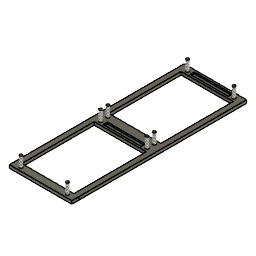
bus (Autodesk Fusion 360 archive; units mm, degrees)
design "ramka na 2 ekrany"
part number: 2026-03-25-11-53-01-845
Autodesk Fusion 360 part; units mm, degrees
note: some values were not read from the file. Chosen so that the rebuilt part matches the saved one: which bodies a step acts on; which face or edge a step refers to; how an offset face is resized. Set by a fixed rule: which sketch regions a step uses.
sketch "Sketch1" plane through (0, 0, 0) normal (0, 0, 1) x (1, 0, 0)
  line L0 (45, 35) -> (-45, 35)
  line L1 (-45, 35) -> (-45, -35)
  line L2 (-45, -35) -> (45, -35)
  line L3 (45, -35) -> (45, 35)
  line L4 (45, 35) -> (-45, -35) construction
  line L5 (-45, 35) -> (45, -35) construction
  line L6 (34.75, 25.0029) -> (-34.75, 25.0029)
  line L7 (-34.75, 25.0029) -> (-34.75, -24.9971)
  line L8 (-34.75, -24.9971) -> (34.75, -24.9971)
  line L9 (34.75, -24.9971) -> (34.75, 25.0029)
  line L10 (34.75, 25.0029) -> (-34.75, -24.9971) construction
  line L11 (-34.75, 25.0029) -> (34.75, -24.9971) construction
  point P0 (0, 0.0029)
  dimension "d1" = 90
  dimension "d2" = 70
  dimension "d3" = 69.5
  dimension "d4" = 50
  constraint horizontal L0
  constraint perpendicular L0 L1
  constraint parallel L0 L2
  constraint parallel L1 L3
  constraint coincident L4 origin
  constraint coincident L5 origin
  constraint horizontal L6
  constraint perpendicular L6 L7
  constraint parallel L6 L8
  constraint parallel L7 L9
  constraint coincident L10 P0
  constraint coincident L11 P0
  measures "d1" distance of L0.start L0.end
  measures "d2" distance of L0.start L2.end
  measures "d3" distance of L6.start L6.end
  measures "d4" distance of L6.start L8.end
extrude "Extrude1" add sketch "Sketch1" along normal blind 3 contours L0 L1 L2 L3 | L6 L7 L8 L9 makes body 1
extrude "Extrude2" cut sketch "Sketch1" along normal blind 42 contours L6 L7 L8 L9 bodies 1
ref_plane "WorkPlane1" through (0, 0, 3) normal (0, 0, 1) x (1, 0, 0)
sketch "Sketch2" plane through (0, 0, 3) normal (0, 0, 1) x (1, 0, 0)
  line L0 (38.25, 22.5) -> (38.25, 22.8)
  line L1 (38.25, 22.8) -> (38.25, 27.2)
  line L2 (38.25, 27.2) -> (38.25, -28)
  line L3 (34.7, 25) -> (34.8, 25)
  line L4 (38.25, 25) -> (38.25, 23.8)
  line L5 (34.7, -25) -> (40.2, -25)
  line L6 (38.25, -25) -> (38.25, -23.8)
  circle A0 centre (38.2495, -22.3) radius 1.5
  line L7 (34.8, 25) -> (39.15, 25)
  line L8 (38.25, 25) -> (38.25, 23.8)
  circle A1 centre (38.25, 22.3) radius 1.5
  line L9 (-34, -25) -> (-44, -25)
  line L10 (-22, 25) -> (-43.5908, 25)
  line L11 (-34.75, 25) -> (-38.25, 25)
  line L12 (-38.25, 25) -> (-38.25, -25)
  line L13 (-38.25, -25) -> (-38.25, -23.8)
  circle A2 centre (-38.25, -22.3041) radius 1.5
  line L14 (-38.25, 25) -> (-38.25, 23.8)
  circle A3 centre (-38.25, 22.2805) radius 1.5
  dimension "d13" = 1.2
  dimension "d14" = 3
  dimension "d15" = 1.2
  dimension "d16" = 3
  dimension "d17" = 3.5
  dimension "d18" = 1.2
  dimension "d19" = 3
  dimension "d20" = 1.2
  dimension "d21" = 3
  constraint perpendicular L2 L3
  constraint midpoint L1 L4.start
  constraint perpendicular L2 L5
  constraint coincident L5 L6.start
  constraint coincident L2 L6.start
  constraint perpendicular L5 L6
  constraint coincident L6.end A0
  constraint parallel L3 L7
  constraint coincident L1 A1.centre
  constraint horizontal L9
  constraint horizontal L10
  constraint coincident L10 L11.start
  constraint parallel L10 L11
  constraint coincident L9 L12.end
  constraint perpendicular L9 L12
  constraint perpendicular L9 L13
  constraint coincident L12 A2.centre
  constraint perpendicular L10 L14
  constraint coincident L12 A3.centre
  measures "d13" distance of L6.start L6.end
  measures "d14" diameter of A0
  measures "d15" distance of L4.start L4.end
  measures "d16" diameter of A1
  measures "d17" distance of L11.start L11.end
  measures "d18" distance of L12.end L13.end
  measures "d19" diameter of A2
  measures "d20" distance of L11.end L14.end
  measures "d21" diameter of A3
extrude "Extrude3" add sketch "Sketch2" along normal blind 10 separate body contours L12 A3 | L12 A3 makes body 2
thread "Thread1" "ISO Metric profile 3.0 M3x0.5 M3x0.5 6g" major diameter 2.927 minor diameter 2.3555 pitch 0.5 angle 60 resizes the face on face at (-37.0709, 23.2078, 9.6667) on bodies 2
extrude "Extrude4" add sketch "Sketch2" along normal blind 10 separate body contours L0 L1 L2 A1 | L0 L1 L2 A1 | L2 A0 | L2 A0 | L12 L13 A2 | L12 L13 A2 makes body 3 at (-37.9895, -23.7813, 9.6667) makes body 4 at (37.5652, -20.9652, 9.6667) makes body 5 at (37.5657, 23.6348, 9.6667)
thread "Thread2" "ISO Metric profile 3.0 M3x0.5 M3x0.5 6g" major diameter 2.927 minor diameter 2.3555 pitch 0.5 angle 60 resizes the face on face at (-37.9895, -23.7813, 9.6667) on face at (37.5652, -20.9652, 9.6667) on face at (37.5657, 23.6348, 9.6667) on bodies 3 4 5
sketch "Sketch3" plane through (0, 0, 0) normal (0, 0, 1) x (1, 0, 0)
  line L0 (-2.8868, 5) -> (-5.7735, 0)
  line L1 (-5.7735, 0) -> (-2.8868, -5)
  line L2 (-2.8868, -5) -> (2.8868, -5)
  line L3 (2.8868, -5) -> (5.7735, 0)
  line L4 (5.7735, 0) -> (2.8868, 5)
  line L5 (2.8868, 5) -> (-2.8868, 5)
  circle A0 centre (0, 0) radius 1.5
  dimension "d30" = 5
  dimension "d31" = 3
  constraint coincident A0.centre origin
  measures "d30" distance of A0.centre L5
  measures "d31" diameter of A0
sketch "Sketch4" plane through (0, 0, 3) normal (0, 0, 1) x (1, 0, 0)
  line L0 (34.75, 0) -> (38.75, 0)
  line L1 (42.75, 0) -> (42.75, -18.25)
  line L2 (42.75, -18.25) -> (38.75, -18.25)
  line L3 (38.75, -18.25) -> (38.75, 0)
  line L4 (38.75, 0) -> (38.75, 18.25)
  line L5 (38.75, 18.25) -> (42.75, 18.25)
  line L6 (42.75, 18.25) -> (42.75, 0)
  dimension "d37" = 4
  dimension "d38" = 18.25
  dimension "d39" = 4
  dimension "d40" = 4
  dimension "d41" = 18.25
  constraint horizontal L0
  constraint vertical L1
  constraint horizontal L2
  constraint vertical L3
  constraint vertical L4
  constraint horizontal L5
  constraint vertical L6
  measures "d37" distance of L0.start L0.end
  measures "d38" distance of L0.end L2.end
  measures "d39" distance of L0.end L1.start
  measures "d40" distance of L1.start L0.end
  measures "d41" distance of L1.start L5.end
extrude "Extrude6" cut sketch "Sketch4" against normal blind 1.5 bodies 1
combine "Combine1" operation add target body 1 tool bodies 2 3 5 4
move_body "Move1" bodies 1 to x (0, 1, 0) y (0, 0, 1) z (1, 0, 0) at (-45, 10, 35)
move_body "Move2" bodies 1 to x (0, 0, 1) y (0, 1, 0) z (-1, 0, 0) at (6.0688, 0, 90.0688)
move_body "Move3" bodies 1 to x (1, 0, 0) y (0, 1, 0) z (0, 0, 1) at (0, 0, -45)
extrude "Extrude7" cut 1 faces at (-22.8478, 48.75, 2.0688) along direction (0, -1, 0) blind 2 on bodies 1 bodies 1
extrude "Extrude8" add 1 faces at (-35.0145, 52.75, 2.0688) along direction (0, -1, 0) blind 1.5 on bodies 1 bodies 1
ref_plane "WorkPlane2" through (-28.9312, 10, 3.0688) normal (0, 0, 1) x (0, 1, 0)
sketch "Sketch5" plane through (0, 0, 3.0688) normal (0, 0, 1) x (1, 0, 0)
  line L0 (-53.9341, 44.75) -> (-3.9341, 44.75)
  line L1 (-3.9341, -24.75) -> (-53.9341, -24.75)
  line L2 (-3.9341, 44.75) -> (-3.9341, -24.75)
  line L3 (-53.9341, -24.75) -> (-53.9341, 44.75)
  line L4 (-31.0518, 51.75) -> (-58.9341, 51.75)
  line L5 (-58.9341, 51.75) -> (-58.9341, 25.022)
  line L6 (-58.9341, 25.022) -> (-58.9341, -31)
  line L7 (-58.9341, -31) -> (-58.9341, -31.75)
  line L8 (-58.9341, -31.75) -> (-30.0627, -31.75)
  line L9 (-30.0627, -31.75) -> (1, -31.75)
  line L10 (1, -31.75) -> (4, -31.75)
  line L11 (1.0659, -24.75) -> (1, -31.75)
  line L12 (1.0659, -24.75) -> (1.0659, 24.1629)
  line L13 (1.0659, 44.75) -> (1.0659, 24.1629)
  line L14 (-31.0518, 51.75) -> (1.0659, 51.75)
  line L15 (1.0659, 51.75) -> (1.0659, 44.75)
  dimension "d54" = 5
  dimension "d55" = 5
  measures "d54" distance of L1.start L11.start
  measures "d55" distance of L0.end L13.start
split "Split1" by curves path "Sketch5" along L11 L12 L13 L15 L14 L4 L5 L6 L7 L8 L9 bodies 1 makes body 6 at (4.4012, 14.721, 3.0688)
delete_body "RemoveBody1" bodies 6
extrude "Extrude9" add 1 faces at (-35.0145, 51.25, 2.0688) along direction (0, -1, 0) blind 0.5 on bodies 1 bodies 1
copy_body "CopyPasteBodies1" bodies 1 makes body 7
move_body "Move4" bodies 7 to x (1, 0, 0) y (0, 1, 0) z (0, 0, 1) at (0, 83.5, 0)
ref_plane "WorkPlane3" through (1.0659, 13.5, 1.5688) normal (1, 0, 0) x (0, 1, 0)
sketch "Sketch6" plane through (1.0659, 0, 0) normal (1, 0, 0) x (0, 1, 0)
  line L0 (51.75, 3.0688) -> (-24.75, 3.0688)
  line L1 (-24.75, 3.0688) -> (-24.75, 0.0688)
  line L2 (-24.75, 0.0688) -> (51.75, 0.0688)
  line L3 (51.75, 0.0688) -> (51.75, 3.0688)
  line L4 (-31.75, 3.0688) -> (135.25, 3.0688)
  line L5 (135.25, 3.0688) -> (135.25, 0.0688)
  line L6 (135.25, 0.0688) -> (-31.75, 0.0688)
  line L7 (-31.75, 0.0688) -> (-31.75, 3.0688)
  point P0 (-31.75, 3.0688)
  point P1 (135.25, 0.0688)
  constraint horizontal L4
  constraint vertical L5
  constraint horizontal L6
  constraint vertical L7
  constraint coincident P1 L5.end
  constraint coincident P0 L4.start
extrude "Extrude10" add sketch "Sketch6" against normal blind 2 contours L3 L4 L5 L6 bodies 1 7
extrude "Extrude11" add 1 faces at (-38.9341, 135.25, 2.0688) along direction (0, 1, 0) blind 1 on bodies 1 bodies 1

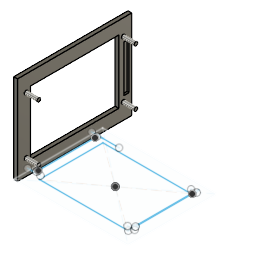
design "ekran TFT"
part number: 2026-03-25-11-53-01-845
Autodesk Fusion 360 part; units mm, degrees
sketch "Sketch1" plane through (0, 0, 0) normal (0, 0, 1) x (1, 0, 0)
  line L0 (45, 35) -> (-45, 35)
  line L1 (-45, 35) -> (-45, -35)
  line L2 (-45, -35) -> (45, -35)
  line L3 (45, -35) -> (45, 35)
  line L4 (45, 35) -> (-45, -35) construction
  line L5 (-45, 35) -> (45, -35) construction
  line L6 (34.75, 25.0029) -> (-34.75, 25.0029)
  line L7 (-34.75, 25.0029) -> (-34.75, -24.9971)
  line L8 (-34.75, -24.9971) -> (34.75, -24.9971)
  line L9 (34.75, -24.9971) -> (34.75, 25.0029)
  line L10 (34.75, 25.0029) -> (-34.75, -24.9971) construction
  line L11 (-34.75, 25.0029) -> (34.75, -24.9971) construction
  point P0 (0, 0.0029)
  dimension "d1" = 90
  dimension "d2" = 70
  dimension "d3" = 69.5
  dimension "d4" = 50
  constraint horizontal L0
  constraint perpendicular L0 L1
  constraint parallel L0 L2
  constraint parallel L1 L3
  constraint coincident L4 origin
  constraint coincident L5 origin
  constraint horizontal L6
  constraint perpendicular L6 L7
  constraint parallel L6 L8
  constraint parallel L7 L9
  constraint coincident L10 P0
  constraint coincident L11 P0
  measures "d1" distance of L0.start L0.end
  measures "d2" distance of L0.start L2.end
  measures "d3" distance of L6.start L6.end
  measures "d4" distance of L6.start L8.end
extrude "Extrude1" add sketch "Sketch1" along normal blind 3 contours L0 L1 L2 L3 | L6 L7 L8 L9 makes body 1
extrude "Extrude2" cut sketch "Sketch1" along normal blind 42 contours L6 L7 L8 L9 bodies 1
ref_plane "WorkPlane1" through (0, 0, 3) normal (0, 0, 1) x (1, 0, 0)
sketch "Sketch2" plane through (0, 0, 3) normal (0, 0, 1) x (1, 0, 0)
  line L0 (38.25, 22.5) -> (38.25, 22.8)
  line L1 (38.25, 22.8) -> (38.25, 27.2)
  line L2 (38.25, 27.2) -> (38.25, -28)
  line L3 (34.7, 25) -> (34.8, 25)
  line L4 (38.25, 25) -> (38.25, 23.8)
  line L5 (34.7, -25) -> (40.2, -25)
  line L6 (38.25, -25) -> (38.25, -23.8)
  circle A0 centre (38.2495, -22.3) radius 1.5
  line L7 (34.8, 25) -> (39.15, 25)
  line L8 (38.25, 25) -> (38.25, 23.8)
  circle A1 centre (38.25, 22.3) radius 1.5
  line L9 (-34, -25) -> (-44, -25)
  line L10 (-22, 25) -> (-43.5908, 25)
  line L11 (-34.75, 25) -> (-38.25, 25)
  line L12 (-38.25, 25) -> (-38.25, -25)
  line L13 (-38.25, -25) -> (-38.25, -23.8)
  circle A2 centre (-38.25, -22.3041) radius 1.5
  line L14 (-38.25, 25) -> (-38.25, 23.8)
  circle A3 centre (-38.25, 22.2805) radius 1.5
  dimension "d13" = 1.2
  dimension "d14" = 3
  dimension "d15" = 1.2
  dimension "d16" = 3
  dimension "d17" = 3.5
  dimension "d18" = 1.2
  dimension "d19" = 3
  dimension "d20" = 1.2
  dimension "d21" = 3
  constraint perpendicular L2 L3
  constraint midpoint L1 L4.start
  constraint perpendicular L2 L5
  constraint coincident L5 L6.start
  constraint coincident L2 L6.start
  constraint perpendicular L5 L6
  constraint coincident L6.end A0
  constraint parallel L3 L7
  constraint coincident L1 A1.centre
  constraint horizontal L9
  constraint horizontal L10
  constraint coincident L10 L11.start
  constraint parallel L10 L11
  constraint coincident L9 L12.end
  constraint perpendicular L9 L12
  constraint perpendicular L9 L13
  constraint coincident L12 A2.centre
  constraint perpendicular L10 L14
  constraint coincident L12 A3.centre
  measures "d13" distance of L6.start L6.end
  measures "d14" diameter of A0
  measures "d15" distance of L4.start L4.end
  measures "d16" diameter of A1
  measures "d17" distance of L11.start L11.end
  measures "d18" distance of L12.end L13.end
  measures "d19" diameter of A2
  measures "d20" distance of L11.end L14.end
  measures "d21" diameter of A3
extrude "Extrude3" add sketch "Sketch2" along normal blind 10 separate body contours L12 A3 | L12 A3 makes body 2
thread "Thread1" "ISO Metric profile 3.0 M3x0.5 M3x0.5 6g" major diameter 2.927 minor diameter 2.3555 pitch 0.5 angle 60 resizes the face on face at (-37.0709, 23.2078, 9.6667) on bodies 2
extrude "Extrude4" add sketch "Sketch2" along normal blind 10 separate body contours L0 L1 L2 A1 | L0 L1 L2 A1 | L2 A0 | L2 A0 | L12 L13 A2 | L12 L13 A2 makes body 3 at (-37.9895, -23.7813, 9.6667) makes body 4 at (37.5652, -20.9652, 9.6667) makes body 5 at (37.5657, 23.6348, 9.6667)
thread "Thread2" "ISO Metric profile 3.0 M3x0.5 M3x0.5 6g" major diameter 2.927 minor diameter 2.3555 pitch 0.5 angle 60 resizes the face on face at (-37.9895, -23.7813, 9.6667) on face at (37.5652, -20.9652, 9.6667) on face at (37.5657, 23.6348, 9.6667) on bodies 3 4 5
sketch "Sketch3" plane through (0, 0, 0) normal (0, 0, 1) x (1, 0, 0)
  line L0 (-2.8868, 5) -> (-5.7735, 0)
  line L1 (-5.7735, 0) -> (-2.8868, -5)
  line L2 (-2.8868, -5) -> (2.8868, -5)
  line L3 (2.8868, -5) -> (5.7735, 0)
  line L4 (5.7735, 0) -> (2.8868, 5)
  line L5 (2.8868, 5) -> (-2.8868, 5)
  circle A0 centre (0, 0) radius 1.5
  dimension "d30" = 5
  dimension "d31" = 3
  constraint coincident A0.centre origin
  measures "d30" distance of A0.centre L5
  measures "d31" diameter of A0
sketch "Sketch4" plane through (0, 0, 3) normal (0, 0, 1) x (1, 0, 0)
  line L0 (34.75, 0) -> (38.75, 0)
  line L1 (42.75, 0) -> (42.75, -18.25)
  line L2 (42.75, -18.25) -> (38.75, -18.25)
  line L3 (38.75, -18.25) -> (38.75, 0)
  line L4 (38.75, 0) -> (38.75, 18.25)
  line L5 (38.75, 18.25) -> (42.75, 18.25)
  line L6 (42.75, 18.25) -> (42.75, 0)
  dimension "d37" = 4
  dimension "d38" = 18.25
  dimension "d39" = 4
  dimension "d40" = 4
  dimension "d41" = 18.25
  constraint horizontal L0
  constraint vertical L1
  constraint horizontal L2
  constraint vertical L3
  constraint vertical L4
  constraint horizontal L5
  constraint vertical L6
  measures "d37" distance of L0.start L0.end
  measures "d38" distance of L0.end L2.end
  measures "d39" distance of L0.end L1.start
  measures "d40" distance of L1.start L0.end
  measures "d41" distance of L1.start L5.end
extrude "Extrude6" cut sketch "Sketch4" against normal blind 1.5 bodies 1
combine "Combine1" operation add target body 1 tool bodies 2 3 5 4
move_body "Move1" bodies 1 to x (0, 1, 0) y (0, 0, 1) z (1, 0, 0) at (-45, 10, 35)

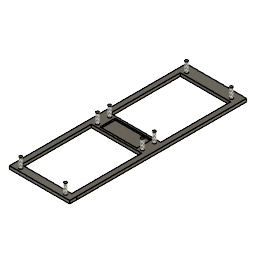
design "ramka wersja 4327643276"
part number: 2026-03-25-11-53-01-845
Autodesk Fusion 360 part; units mm, degrees
sketch "Sketch1" plane through (0, 0, 0) normal (0, 0, 1) x (1, 0, 0)
  line L0 (45, 35) -> (-45, 35)
  line L1 (-45, 35) -> (-45, -35)
  line L2 (-45, -35) -> (45, -35)
  line L3 (45, -35) -> (45, 35)
  line L4 (45, 35) -> (-45, -35) construction
  line L5 (-45, 35) -> (45, -35) construction
  line L6 (34.75, 25.0029) -> (-34.75, 25.0029)
  line L7 (-34.75, 25.0029) -> (-34.75, -24.9971)
  line L8 (-34.75, -24.9971) -> (34.75, -24.9971)
  line L9 (34.75, -24.9971) -> (34.75, 25.0029)
  line L10 (34.75, 25.0029) -> (-34.75, -24.9971) construction
  line L11 (-34.75, 25.0029) -> (34.75, -24.9971) construction
  point P0 (0, 0.0029)
  dimension "d1" = 90
  dimension "d2" = 70
  dimension "d3" = 69.5
  dimension "d4" = 50
  constraint horizontal L0
  constraint perpendicular L0 L1
  constraint parallel L0 L2
  constraint parallel L1 L3
  constraint coincident L4 origin
  constraint coincident L5 origin
  constraint horizontal L6
  constraint perpendicular L6 L7
  constraint parallel L6 L8
  constraint parallel L7 L9
  constraint coincident L10 P0
  constraint coincident L11 P0
  measures "d1" distance of L0.start L0.end
  measures "d2" distance of L0.start L2.end
  measures "d3" distance of L6.start L6.end
  measures "d4" distance of L6.start L8.end
extrude "Extrude1" add sketch "Sketch1" along normal blind 3 contours L0 L1 L2 L3 | L6 L7 L8 L9 makes body 1
extrude "Extrude2" cut sketch "Sketch1" along normal blind 42 contours L6 L7 L8 L9 bodies 1
ref_plane "WorkPlane1" through (0, 0, 3) normal (0, 0, 1) x (1, 0, 0)
sketch "Sketch2" plane through (0, 0, 3) normal (0, 0, 1) x (1, 0, 0)
  line L0 (38.25, 22.5) -> (38.25, 22.8)
  line L1 (38.25, 22.8) -> (38.25, 27.2)
  line L2 (38.25, 27.2) -> (38.25, -28)
  line L3 (34.7, 25) -> (34.8, 25)
  line L4 (38.25, 25) -> (38.25, 23.8)
  line L5 (34.7, -25) -> (40.2, -25)
  line L6 (38.25, -25) -> (38.25, -23.8)
  circle A0 centre (38.2495, -22.3) radius 1.5
  line L7 (34.8, 25) -> (39.15, 25)
  line L8 (38.25, 25) -> (38.25, 23.8)
  circle A1 centre (38.25, 22.3) radius 1.5
  line L9 (-34, -25) -> (-44, -25)
  line L10 (-22, 25) -> (-43.5908, 25)
  line L11 (-34.75, 25) -> (-38.25, 25)
  line L12 (-38.25, 25) -> (-38.25, -25)
  line L13 (-38.25, -25) -> (-38.25, -23.8)
  circle A2 centre (-38.25, -22.3041) radius 1.5
  line L14 (-38.25, 25) -> (-38.25, 23.8)
  circle A3 centre (-38.25, 22.2805) radius 1.5
  dimension "d13" = 1.2
  dimension "d14" = 3
  dimension "d15" = 1.2
  dimension "d16" = 3
  dimension "d17" = 3.5
  dimension "d18" = 1.2
  dimension "d19" = 3
  dimension "d20" = 1.2
  dimension "d21" = 3
  constraint perpendicular L2 L3
  constraint midpoint L1 L4.start
  constraint perpendicular L2 L5
  constraint coincident L5 L6.start
  constraint coincident L2 L6.start
  constraint perpendicular L5 L6
  constraint coincident L6.end A0
  constraint parallel L3 L7
  constraint coincident L1 A1.centre
  constraint horizontal L9
  constraint horizontal L10
  constraint coincident L10 L11.start
  constraint parallel L10 L11
  constraint coincident L9 L12.end
  constraint perpendicular L9 L12
  constraint perpendicular L9 L13
  constraint coincident L12 A2.centre
  constraint perpendicular L10 L14
  constraint coincident L12 A3.centre
  measures "d13" distance of L6.start L6.end
  measures "d14" diameter of A0
  measures "d15" distance of L4.start L4.end
  measures "d16" diameter of A1
  measures "d17" distance of L11.start L11.end
  measures "d18" distance of L12.end L13.end
  measures "d19" diameter of A2
  measures "d20" distance of L11.end L14.end
  measures "d21" diameter of A3
extrude "Extrude3" add sketch "Sketch2" along normal blind 10 separate body contours L12 A3 | L12 A3 makes body 2
thread "Thread1" "ISO Metric profile 3.0 M3x0.5 M3x0.5 6g" major diameter 2.927 minor diameter 2.3555 pitch 0.5 angle 60 resizes the face on face at (-37.0709, 23.2078, 9.6667) on bodies 2
extrude "Extrude4" add sketch "Sketch2" along normal blind 10 separate body contours L0 L1 L2 A1 | L0 L1 L2 A1 | L2 A0 | L2 A0 | L12 L13 A2 | L12 L13 A2 makes body 3 at (-37.9895, -23.7813, 9.6667) makes body 4 at (37.5652, -20.9652, 9.6667) makes body 5 at (37.5657, 23.6348, 9.6667)
thread "Thread2" "ISO Metric profile 3.0 M3x0.5 M3x0.5 6g" major diameter 2.927 minor diameter 2.3555 pitch 0.5 angle 60 resizes the face on face at (-37.9895, -23.7813, 9.6667) on face at (37.5652, -20.9652, 9.6667) on face at (37.5657, 23.6348, 9.6667) on bodies 3 4 5
sketch "Sketch3" plane through (0, 0, 0) normal (0, 0, 1) x (1, 0, 0)
  line L0 (-2.8868, 5) -> (-5.7735, 0)
  line L1 (-5.7735, 0) -> (-2.8868, -5)
  line L2 (-2.8868, -5) -> (2.8868, -5)
  line L3 (2.8868, -5) -> (5.7735, 0)
  line L4 (5.7735, 0) -> (2.8868, 5)
  line L5 (2.8868, 5) -> (-2.8868, 5)
  circle A0 centre (0, 0) radius 1.5
  dimension "d30" = 5
  dimension "d31" = 3
  constraint coincident A0.centre origin
  measures "d30" distance of A0.centre L5
  measures "d31" diameter of A0
sketch "Sketch4" plane through (0, 0, 3) normal (0, 0, 1) x (1, 0, 0)
  line L0 (34.75, 0) -> (38.75, 0)
  line L1 (42.75, 0) -> (42.75, -18.25)
  line L2 (42.75, -18.25) -> (38.75, -18.25)
  line L3 (38.75, -18.25) -> (38.75, 0)
  line L4 (38.75, 0) -> (38.75, 18.25)
  line L5 (38.75, 18.25) -> (42.75, 18.25)
  line L6 (42.75, 18.25) -> (42.75, 0)
  dimension "d37" = 4
  dimension "d38" = 18.25
  dimension "d39" = 4
  dimension "d40" = 4
  dimension "d41" = 18.25
  constraint horizontal L0
  constraint vertical L1
  constraint horizontal L2
  constraint vertical L3
  constraint vertical L4
  constraint horizontal L5
  constraint vertical L6
  measures "d37" distance of L0.start L0.end
  measures "d38" distance of L0.end L2.end
  measures "d39" distance of L0.end L1.start
  measures "d40" distance of L1.start L0.end
  measures "d41" distance of L1.start L5.end
extrude "Extrude6" cut sketch "Sketch4" against normal blind 1.5 bodies 1
combine "Combine1" operation add target body 1 tool bodies 2 3 5 4
move_body "Move1" bodies 1 to x (0, 1, 0) y (0, 0, 1) z (1, 0, 0) at (-45, 10, 35)
move_body "Move2" bodies 1 to x (0, 0, 1) y (0, 1, 0) z (-1, 0, 0) at (6.0688, 0, 90.0688)
move_body "Move3" bodies 1 to x (1, 0, 0) y (0, 1, 0) z (0, 0, 1) at (0, 0, -45)
extrude "Extrude7" cut 1 faces at (-22.8478, 48.75, 2.0688) along direction (0, -1, 0) blind 2 on bodies 1 bodies 1
extrude "Extrude8" add 1 faces at (-35.0145, 52.75, 2.0688) along direction (0, -1, 0) blind 1.5 on bodies 1 bodies 1
ref_plane "WorkPlane2" through (-28.9312, 10, 3.0688) normal (0, 0, 1) x (0, 1, 0)
sketch "Sketch5" plane through (0, 0, 3.0688) normal (0, 0, 1) x (1, 0, 0)
  line L0 (-53.9341, 44.75) -> (-3.9341, 44.75)
  line L1 (-3.9341, -24.75) -> (-53.9341, -24.75)
  line L2 (-3.9341, 44.75) -> (-3.9341, -24.75)
  line L3 (-53.9341, -24.75) -> (-53.9341, 44.75)
  line L4 (-31.0518, 51.75) -> (-58.9341, 51.75)
  line L5 (-58.9341, 51.75) -> (-58.9341, 25.022)
  line L6 (-58.9341, 25.022) -> (-58.9341, -31)
  line L7 (-58.9341, -31) -> (-58.9341, -31.75)
  line L8 (-58.9341, -31.75) -> (-30.0627, -31.75)
  line L9 (-30.0627, -31.75) -> (1, -31.75)
  line L10 (1, -31.75) -> (4, -31.75)
  line L11 (1.0659, -24.75) -> (1, -31.75)
  line L12 (1.0659, -24.75) -> (1.0659, 24.1629)
  line L13 (1.0659, 44.75) -> (1.0659, 24.1629)
  line L14 (-31.0518, 51.75) -> (1.0659, 51.75)
  line L15 (1.0659, 51.75) -> (1.0659, 44.75)
  dimension "d54" = 5
  dimension "d55" = 5
  measures "d54" distance of L1.start L11.start
  measures "d55" distance of L0.end L13.start
split "Split1" by curves path "Sketch5" along L11 L12 L13 L15 L14 L4 L5 L6 L7 L8 L9 bodies 1 makes body 6 at (4.4012, 14.721, 3.0688)
delete_body "RemoveBody1" bodies 6
extrude "Extrude9" add 1 faces at (-35.0145, 51.25, 2.0688) along direction (0, -1, 0) blind 0.5 on bodies 1 bodies 1
copy_body "CopyPasteBodies1" bodies 1 makes body 7
move_body "Move4" bodies 7 to x (1, 0, 0) y (0, 1, 0) z (0, 0, 1) at (0, 83.5, 0)
ref_plane "WorkPlane3" through (1.0659, 13.5, 1.5688) normal (1, 0, 0) x (0, 1, 0)
sketch "Sketch6" plane through (1.0659, 0, 0) normal (1, 0, 0) x (0, 1, 0)
  line L0 (51.75, 3.0688) -> (-24.75, 3.0688)
  line L1 (-24.75, 3.0688) -> (-24.75, 0.0688)
  line L2 (-24.75, 0.0688) -> (51.75, 0.0688)
  line L3 (51.75, 0.0688) -> (51.75, 3.0688)
  line L4 (-31.75, 3.0688) -> (135.25, 3.0688)
  line L5 (135.25, 3.0688) -> (135.25, 0.0688)
  line L6 (135.25, 0.0688) -> (-31.75, 0.0688)
  line L7 (-31.75, 0.0688) -> (-31.75, 3.0688)
  point P0 (-31.75, 3.0688)
  point P1 (135.25, 0.0688)
  constraint horizontal L4
  constraint vertical L5
  constraint horizontal L6
  constraint vertical L7
  constraint coincident P1 L5.end
  constraint coincident P0 L4.start
extrude "Extrude10" add sketch "Sketch6" against normal blind 2 contours L3 L4 L5 L6 bodies 1 7
extrude "Extrude11" add 1 faces at (-38.9341, 135.25, 2.0688) along direction (0, 1, 0) blind 1 on bodies 1 bodies 1
split "Split2" by plane through (-28.9312, 50.75, 2.3188) normal (0, -1, 0) bodies 1 makes body 8 at (-37.2894, -29.4167, 0.0688)
move_body "Move5" bodies 1 to x (1, 0, 0) y (0, 1, 0) z (0, 0, 1) at (0, 5, 0)
extrude "Extrude12" add 2 faces at (-55.0165, 55.75, 1.5688) (-35.0145, 55.75, 2.5688) along direction (0, -1, 0) blind 5 on bodies 1 bodies 1 8
sketch "Sketch7" plane through (0, 0, 3.0688) normal (0, 0, 1) x (-1, 0, 0)
  line L0 (3.9341, -44.75) -> (3.9341, 24.75)
  line L1 (3.9341, 24.75) -> (53.9341, 24.75)
  line L2 (53.9341, 24.75) -> (53.9341, -44.75)
  line L3 (53.9341, -44.75) -> (3.9341, -44.75)
  circle A0 centre (51.2117, 28.25) radius 1.4635
  circle A1 centre (6.6271, 28.25) radius 1.4635
  circle A2 centre (51.2312, -48.25) radius 1.4635
  circle A3 centre (6.6312, -48.2495) radius 1.4635
  line L4 (47.1812, -50.75) -> (10.6812, -50.75)
  line L5 (10.6812, -50.75) -> (10.6812, -46.75)
  line L6 (10.6812, -46.75) -> (47.1812, -46.75)
  line L7 (47.1812, -46.75) -> (47.1812, -50.75)
  line L8 (47.1812, -135.25) -> (47.1812, -139.25)
  line L9 (47.1812, -139.25) -> (10.6812, -139.25)
  line L10 (10.6812, -139.25) -> (10.6812, -135.25)
  line L11 (10.6812, -135.25) -> (47.1812, -135.25)
  circle A4 centre (6.6312, -136.7495) radius 1.4635
  circle A5 centre (51.2312, -136.75) radius 1.4635
  circle A6 centre (6.6271, -60.25) radius 1.4635
  circle A7 centre (51.2117, -60.25) radius 1.4635
  line L12 (3.9341, -133.25) -> (3.9341, -63.75)
  line L13 (3.9341, -63.75) -> (53.9341, -63.75)
  line L14 (53.9341, -63.75) -> (53.9341, -133.25)
  line L15 (53.9341, -133.25) -> (3.9341, -133.25)
  line L16 (-1.0659, 24.75) -> (-1.0659, -141.25)
  line L17 (-1.0659, -141.25) -> (58.9341, -141.25)
  line L18 (58.9341, -141.25) -> (58.9341, 31.75)
  line L19 (58.9341, 31.75) -> (-1, 31.75)
  line L20 (-1, 31.75) -> (-1.0659, 24.75)
  line L21 (10.6812, -46.75) -> (47.1812, -46.75)
  line L22 (53.9341, -44.75) -> (3.9341, -44.75)
  line L23 (3.9341, -63.75) -> (53.9341, -63.75)
  line L24 (20.1427, -63.75) -> (20.1427, -61.75)
  line L25 (20.1427, -61.75) -> (7.6341, -61.75)
  line L26 (7.6341, -61.75) -> (48, -61.75)
  line L27 (47.1812, -46.75) -> (47.1812, -50.75)
  line L28 (10.6812, -50.75) -> (10.6812, -46.75)
  line L29 (47.1812, -50.75) -> (47.1812, -61.75)
  line L30 (10.6812, -50.75) -> (10.6812, -61)
  line L31 (10.6812, -61) -> (10.6812, -61.75)
  line L32 (10.6812, -50.75) -> (47.1812, -50.75)
  dimension "d66" = 2
  dimension "d67" = 180
  constraint coincident L23 L24.start
  constraint perpendicular L13 L24
  constraint perpendicular L24 L25
  constraint parallel L25 L26
  constraint coincident L4.start L7.end
  constraint coincident L26 L29.end
  constraint perpendicular L26 L29
  constraint coincident L4.end L5.start
  constraint perpendicular L26 L30
  constraint coincident L25 L31.end
  measures "d66" distance of L24.start L24.end
  measures "d67" angle of L30 L31
extrude "Extrude13" cut sketch "Sketch7" against normal blind 1.5 contours L4 L25 L26 L29 L30 L31 L32 bodies 1
extrude "Extrude14" add 1 faces at (-22.8478, 137.9167, 1.5688) along direction (0, 0, 1) blind 1.5 on bodies 1 bodies 1
extrude "Extrude15" add 1 faces at (-38.9341, 141.25, 2.0688) along direction (0, 1, 0) blind 3 on bodies 1 bodies 1
